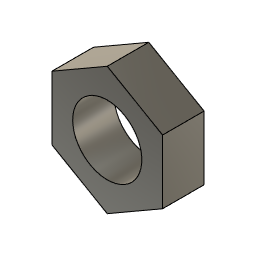
螺母M5 薄款 v1 (Autodesk Fusion 360 design; units mm, degrees)
Autodesk Fusion 360 part; units mm, degrees
sketch "草图1" plane through (0, 0, 0) normal (0, 1, 0) x (1, 0, 0)
  line L0 (0, 0) -> (0, -4.6188)
  line L1 (0, -4.6188) -> (4, -6.9282)
  line L2 (4, -6.9282) -> (8, -4.6188)
  line L3 (8, -4.6188) -> (8, 0)
  line L4 (8, 0) -> (4, 2.3094)
  line L5 (4, 2.3094) -> (0, 0)
  circle A0 centre (4, -2.3094) radius 2.5
  point P0 (4, -2.3094)
  dimension "d2" = 8
  dimension "d3" = 5
  constraint coincident L0.start L5.end
  constraint coincident P0 A0.centre
  measures "d2" distance of L0 L3
  measures "d3" diameter of A0
extrude "拉伸1" add sketch "草图1" along normal blind 3
